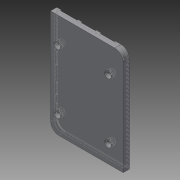
# Autodesk Inventor part: bottom
Saved by Autodesk Inventor 2015 (Build 190159000, 159)
## iProperties
Created: 2015-03-24
Part Number: bottom
Material: Generic
Document SubType Name: Modeling
Designer: Pablo
Density: 1 g/cm^3
Appearance: Default
Author: Pablo
Autodesk Inventor part; units mm, degrees
ref_plane "YZ Plane" through (0, 0, 0) normal (1, 0, 0) x (0, 1, 0)
ref_plane "XZ Plane" through (0, 0, 0) normal (0, 1, 0) x (-1, 0, 0)
ref_plane "XY Plane" through (0, 0, 0) normal (0, 0, 1) x (1, 0, 0)
sketch "base" plane through (0, 0, 0) normal (0, 1, 0) x (-1, 0, 0)
  line L0 (35, 50) -> (-35, 50)
  line L1 (-35, 50) -> (-35, -50)
  line L2 (-35, -50) -> (35, -50)
  line L3 (35, -50) -> (35, 50)
  point P0 (0, 0)
  point P1 (0, 0)
  dimension "d0" = 70
  dimension "d1" = 100
  dimension "d2" = 50
  dimension "d3" = 35
  dimension "d4" = 0
  dimension "d5" = 0
  constraints: 8 end point, 2 parallel, 1 horizontal, 1 perpendicular
  measures "d0" distance of L2.end L1.end
  measures "d1" distance of L1.end L0.end
  measures "d2" distance from line of L2 point (0, 0)
  measures "d3" distance from line of L3 point (0, 0)
  measures "d4" distance of point (0, 0) point (0, 0)
  measures "d5" distance of point (0, 0) point (0, 0)
extrude "baseBody" add sketch "base" along normal blind 5
fillet "filletBaseBody" radius 8 2 edges at (-35, 2.5, -50) (35, 2.5, 50)
shell "shellBaseBody" thickness 2 removed faces 1 at (11.6667, 5, -16.6667)
sketch "baseBorderCase" plane through (0, 5, 0) normal (0, 1, 0) x (1, 0, 0)
  line L0 (-35, -50) -> (27, -50)
  line L1 (35, -42) -> (35, 50)
  line L2 (35, 50) -> (-27, 50)
  line L3 (-35, 42) -> (-35, -50)
  arc A0 (-27, 50) -> (-35, 42) centre (-27, 42) ccw
  arc A1 (27, -50) -> (35, -42) centre (27, -42) ccw
  line L4 (-34, -49) -> (27, -49)
  arc A2 (27, -49) -> (34, -42) centre (27, -42) ccw
  line L5 (34, -42) -> (34, 49)
  line L6 (34, 49) -> (-27, 49)
  arc A3 (-27, 49) -> (-34, 42) centre (-27, 42) ccw
  line L7 (-34, 42) -> (-34, -49)
  point P0 (0, 0)
  dimension "d10" = 8
  dimension "d11" = 1
  constraints: 16 end point, 8 point on circle, 4 centre point, 4 parallel, 4 tangent, 2 perpendicular, 1 equal radius, 1 horizontal, 5 other
  measures "d10" radius of A0
  measures "d11" distance between parallel lines of L3 L7
extrude "borderCase" add sketch "baseBorderCase" along normal blind 1
sketch "baseFrontHoles" plane through (-35, 0, 50) normal (0, 0, 1) x (1, 0, 0)
  line L0 (2, 2) -> (2, 5)
  line L1 (2, 2) -> (2, 5) projected
  line L2 (2, 5) -> (4.5, 5)
  line L3 (4.5, 5) -> (4.5, 18.5)
  line L4 (4.5, 18.5) -> (20.5, 18.5)
  line L5 (20.5, 18.5) -> (20.5, 5)
  line L6 (20.5, 5) -> (4.5, 5)
  line L7 (20.5, 5) -> (24.5, 5)
  line L8 (24.5, 5) -> (24.5, 19.5)
  line L9 (24.5, 19.5) -> (38, 19.5)
  line L10 (38, 19.5) -> (38, 5)
  line L11 (38, 5) -> (24.5, 5)
  line L12 (38, 5) -> (43, 5)
  line L13 (43, 5) -> (43, 19.5)
  line L14 (43, 19.5) -> (56.5, 19.5)
  line L15 (56.5, 19.5) -> (56.5, 5)
  line L16 (56.5, 5) -> (43, 5)
  point P0 (35, 0)
  dimension "d14" = 3
  dimension "d15" = 2.5
  dimension "d16" = 13.5
  dimension "d17" = 16
  dimension "d18" = 13.5
  dimension "d19" = 16
  dimension "d20" = 4
  dimension "d21" = 14.5
  dimension "d22" = 13.5
  dimension "d23" = 14.5
  dimension "d24" = 13.5
  dimension "d25" = 5
  dimension "d26" = 14.5
  dimension "d27" = 13.5
  dimension "d28" = 14.5
  constraints: 32 end point, 7 perpendicular, 3 point on line, 2 horizontal, 1 collinear, 1 vertical
  measures "d14" distance of L0.start L0.end
  measures "d15" distance of L0.end L2.end
  measures "d16" distance of L2.end L3.end
  measures "d17" distance of L3.end L4.end
  measures "d18" distance of L4.end L5.end
  measures "d19" distance of L5.end L2.end
  measures "d20" distance of L5.end L7.end
  measures "d21" distance of L7.end L8.end
  measures "d22" distance of L8.end L9.end
  measures "d23" distance of L9.end L10.end
  measures "d24" distance of L10.end L7.end
  measures "d25" distance of L10.end L12.end
  measures "d26" distance of L12.end L13.end
  measures "d27" distance of L13.end L14.end
  measures "d28" distance of L14.end L15.end
extrude "frontHoles" cut sketch "baseFrontHoles" against normal up to surface (2 mm away)
sketch "baseLateralHoles" plane through (-35, 0, -42) normal (-1, 0, 0) x (0, 0, 1)
  line L0 (90, 2) -> (90, 5)
  line L1 (90, 2) -> (90, 5) projected
  line L2 (90, 5) -> (62.5, 5)
  line L3 (62.5, 5) -> (62.5, 11)
  line L4 (62.5, 11) -> (55.5, 11)
  line L5 (55.5, 11) -> (55.5, 5)
  line L6 (55.5, 5) -> (62.5, 5)
  line L7 (55.5, 5) -> (45, 5)
  line L8 (45, 5) -> (45, 11)
  line L9 (45, 11) -> (30, 11)
  line L10 (30, 11) -> (30, 5)
  line L11 (30, 5) -> (45, 5)
  line L12 (30, 5) -> (20, 5)
  line L13 (20, 5) -> (20, 8)
  line L14 (20, 8) -> (12.5, 8)
  line L15 (12.5, 8) -> (12.5, 5)
  line L16 (12.5, 5) -> (20, 5)
  point P0 (42, 0)
  dimension "d31" = 3
  dimension "d32" = 27.5
  dimension "d33" = 6
  dimension "d34" = 7
  dimension "d35" = 10.5
  dimension "d36" = 6
  dimension "d37" = 15
  dimension "d38" = 10
  dimension "d39" = 3
  dimension "d40" = 7.5
  constraints: 32 end point, 12 perpendicular, 5 point on line, 1 vertical
  measures "d31" distance of L0.start L0.end
  measures "d32" distance of L0.end L2.end
  measures "d33" distance of L2.end L3.end
  measures "d34" distance of L3.end L4.end
  measures "d35" distance of L5.end L7.end
  measures "d36" distance of L7.end L8.end
  measures "d37" distance of L8.end L9.end
  measures "d38" distance of L10.end L12.end
  measures "d39" distance of L12.end L13.end
  measures "d40" distance of L13.end L14.end
extrude "lateralHoles" cut sketch "baseLateralHoles" against normal up to surface (2 mm away)
sketch "baseScrewHolders" plane through (-27, 2, -48) normal (0, 1, 0) x (1, 0, 0)
  line L0 (-1.6495, -96) -> (-1.6495, -72.425)
  circle A0 centre (-1.6495, -72.425) radius 1.25
  line L1 (-1.6495, -72.425) -> (47.3005, -72.425)
  line L2 (47.3005, -72.425) -> (47.3005, -14.925)
  line L3 (47.3005, -14.925) -> (-1.6495, -14.925)
  line L4 (-1.6495, -14.925) -> (-1.6495, -72.425)
  circle A1 centre (47.3005, -72.425) radius 1.25
  circle A2 centre (47.3005, -14.925) radius 1.25
  circle A3 centre (-1.6495, -14.925) radius 1.25
  circle A4 centre (-1.6495, -14.925) radius 3.25
  circle A5 centre (47.3005, -14.925) radius 3.25
  circle A6 centre (47.3005, -72.425) radius 3.25
  circle A7 centre (-1.6495, -72.425) radius 3.25
  point P0 (27, -48)
  point P1 (-6, -96)
  dimension "d44" = 23.575
  dimension "d45" = 2.5
  dimension "d46" = 48.95
  dimension "d47" = 57.5
  dimension "d48" = 2.5
  dimension "d49" = 2.5
  dimension "d50" = 2.5
  dimension "d51" = 6.5
  dimension "d52" = 6.5
  dimension "d53" = 6.5
  dimension "d54" = 6.5
  dimension "d74" = 4.3505
  constraints: 10 end point, 8 centre point, 8 coincident, 2 horizontal, 2 perpendicular, 1 vertical
  measures "d44" distance of L0.start L0.end
  measures "d45" diameter of A0
  measures "d46" distance of L1.start L1.end
  measures "d47" distance of L1.end L2.end
  measures "d48" diameter of A1
  measures "d49" diameter of A2
  measures "d50" diameter of A3
  measures "d51" diameter of A4
  measures "d52" diameter of A5
  measures "d53" diameter of A6
  measures "d54" diameter of A7
  measures "d74" distance from line of L0 point (-6, -96)
extrude "screwHolders" add sketch "baseScrewHolders" along normal blind 3 contours A7 L4 A0 L0 | L0 A0 L1 A7 | A7 L1 A0 L4 | A4 L3 A3 L4 | L4 A3 L3 A4 | A6 L2 A1 L1 | L1 A1 L2 A6 | A5 L2 A2 L3 | L3 A2 L2 A5
extrude "screwHoles" cut sketch "baseScrewHolders" against normal up to next contours A0 L4 L0 | L0 L1 A0 | L4 A0 L1 | A3 L3 L4 | L4 L3 A3 | A1 L2 L1 | L1 L2 A1 | A2 L2 L3 | L3 L2 A2
chamfer "screwHolderChamfler1" distance 3 angle 10 1 edges at (-31.8995, 5, -33.075) measured on face at (-25.41, 4, -32.8135)
chamfer "screwHolderChamfler2" distance 3 angle 10 1 edges at (17.0505, 5, -33.075) measured on face at (23.54, 4, -32.8135)
chamfer "screwHolderChamfler3" distance 3 angle 10 1 edges at (17.0505, 5, 24.425) measured on face at (23.54, 4, 24.6865)
chamfer "screwHolderChamfler4" distance 3 angle 10 1 edges at (-31.8995, 5, 24.425) measured on face at (-25.41, 4, 24.6865)
chamfer "Chamfer5" distance 2 angle 45 4 edges at (19.0505, 0, 24.425) (-29.8995, 0, 24.425) (-29.8995, 0, -33.075) (19.0505, 0, -33.075)
equation "\"d48\" = d45"
equation "\"d49\" = d48"
equation "\"d50\" = d49"
equation "\"d51\" = d52"
equation "\"d52\" = d53"
equation "\"d53\" = d54"
body "Solid1"
